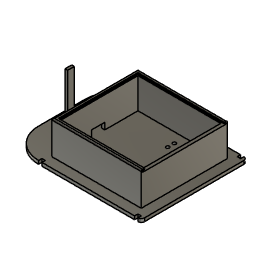
Robot_body (Autodesk Fusion 360 design; units mm, degrees)
Autodesk Fusion 360 part; units mm, degrees
sketch "Szkic1" plane through (0, 0, 0) normal (0, 0, 1) x (1, 0, 0)
  line L0 (100, -80) -> (-100, -80)
  line L1 (-100, -80) -> (-100, 80)
  line L2 (-100, 80) -> (100, 80)
  line L3 (100, 80) -> (100, -80)
  line L4 (100, -80) -> (-100, 80) construction
  line L5 (-100, -80) -> (100, 80) construction
  dimension "d1" = 200
  dimension "d2" = 160
  constraint horizontal L0
  constraint perpendicular L0 L1
  constraint parallel L0 L2
  constraint parallel L1 L3
  constraint coincident L4 origin
  constraint coincident L5 origin
  measures "d1" distance of L1.end L2.end
  measures "d2" distance of L0.end L1.end
extrude "Wyciągnięcie proste1" add sketch "Szkic1" along normal blind 5
sketch "Szkic2" plane through (0, 0, 5) normal (0, 0, 1) x (-1, 0, 0)
  line L0 (-100, -80) -> (100, -80)
  line L1 (100, -80) -> (100, 80)
  line L2 (100, 80) -> (-100, 80)
  line L3 (-100, 80) -> (-100, -80)
  line L4 (-90, 80) -> (-95, 80)
  line L5 (-95, 80) -> (-95, 75)
  line L6 (-95, 75) -> (-90, 75)
  line L7 (-90, 75) -> (-90, 80)
  dimension "d5" = 5
  dimension "d6" = 5
  constraint horizontal L4
  constraint vertical L5
  constraint horizontal L6
  constraint vertical L7
  constraint coincident L2 L4.start
  measures "d5" distance of L4.start L4.end
  measures "d6" distance of L4.start L6.end
extrude "Wyciągnięcie proste2" cut sketch "Szkic2" against normal blind 5 contours L2 L4 L5 L6 L7
sketch "Szkic3" plane through (0, 0, 5) normal (0, 0, 1) x (-1, 0, 0)
  line L0 (-95, 75) -> (-95, 80)
  line L1 (-95, 80) -> (-100, 80)
  line L2 (-100, 80) -> (-100, -80)
  line L3 (-100, -80) -> (100, -80)
  line L4 (100, -80) -> (100, 80)
  line L5 (100, 80) -> (-90, 80)
  line L6 (-90, 80) -> (-90, 75)
  line L7 (-90, 75) -> (-95, 75)
  line L8 (-90, -80) -> (-95, -80)
  line L9 (-95, -80) -> (-95, -75)
  line L10 (-95, -75) -> (-90, -75)
  line L11 (-90, -75) -> (-90, -80)
  dimension "d9" = 5
  dimension "d10" = 5
  constraint horizontal L8
  constraint vertical L9
  constraint horizontal L10
  constraint vertical L11
  constraint coincident L3 L8.start
  measures "d9" distance of L8.start L8.end
  measures "d10" distance of L8.start L10.end
extrude "Wyciągnięcie proste3" cut sketch "Szkic3" against normal blind 5 contours L3 L8 L9 L10 L11
sketch "Szkic4" plane through (0, 0, 5) normal (0, 0, 1) x (-1, 0, 0)
  line L0 (-90, -75) -> (-90, -80)
  line L1 (-90, -80) -> (100, -80)
  line L2 (100, -80) -> (100, 80)
  line L3 (100, 80) -> (-90, 80)
  line L4 (-90, 80) -> (-90, 75)
  line L5 (-90, 75) -> (-95, 75)
  line L6 (-95, 75) -> (-95, 80)
  line L7 (-95, 80) -> (-100, 80)
  line L8 (-100, 80) -> (-100, -80)
  line L9 (-100, -80) -> (-95, -80)
  line L10 (-95, -80) -> (-95, -75)
  line L11 (-95, -75) -> (-90, -75)
  line L12 (50, -80) -> (55, -80)
  line L13 (55, -80) -> (55, -75)
  line L14 (55, -75) -> (50, -75)
  line L15 (50, -75) -> (50, -80)
  dimension "d13" = 5
  dimension "d14" = 5
  constraint horizontal L12
  constraint vertical L13
  constraint horizontal L14
  constraint vertical L15
  constraint coincident L1 L12.start
  measures "d13" distance of L12.start L12.end
  measures "d14" distance of L12.start L14.end
extrude "Wyciągnięcie proste4" cut sketch "Szkic4" against normal blind 5 contours L1 L12 L13 L14 L15
sketch "Szkic5" plane through (0, 0, 5) normal (0, 0, 1) x (-1, 0, 0)
  line L0 (50, -80) -> (50, -75)
  line L1 (50, -75) -> (55, -75)
  line L2 (55, -75) -> (55, -80)
  line L3 (55, -80) -> (100, -80)
  line L4 (100, -80) -> (100, 80)
  line L5 (100, 80) -> (-90, 80)
  line L6 (-90, 80) -> (-90, 75)
  line L7 (-90, 75) -> (-95, 75)
  line L8 (-95, 75) -> (-95, 80)
  line L9 (-95, 80) -> (-100, 80)
  line L10 (-100, 80) -> (-100, -80)
  line L11 (-100, -80) -> (-95, -80)
  line L12 (-95, -80) -> (-95, -75)
  line L13 (-95, -75) -> (-90, -75)
  line L14 (-90, -75) -> (-90, -80)
  line L15 (-90, -80) -> (50, -80)
  line L16 (50, 80) -> (55, 80)
  line L17 (55, 80) -> (55, 75)
  line L18 (55, 75) -> (50, 75)
  line L19 (50, 75) -> (50, 80)
  dimension "d17" = 5
  dimension "d18" = 5
  constraint horizontal L16
  constraint vertical L17
  constraint horizontal L18
  constraint vertical L19
  constraint coincident L5 L16.start
  measures "d17" distance of L16.start L16.end
  measures "d18" distance of L16.start L18.end
extrude "Wyciągnięcie proste5" cut sketch "Szkic5" against normal blind 5 contours L5 L16 L17 L18 L19
sketch "Szkic6" plane through (0, 0, 5) normal (0, 0, 1) x (-1, 0, 0)
  line L0 (50, 75) -> (50, 80)
  line L1 (50, 80) -> (-90, 80)
  line L2 (-90, 80) -> (-90, 75)
  line L3 (-90, 75) -> (-95, 75)
  line L4 (-95, 75) -> (-95, 80)
  line L5 (-95, 80) -> (-100, 80)
  line L6 (-100, 80) -> (-100, -80)
  line L7 (-100, -80) -> (-95, -80)
  line L8 (-95, -80) -> (-95, -75)
  line L9 (-95, -75) -> (-90, -75)
  line L10 (-90, -75) -> (-90, -80)
  line L11 (-90, -80) -> (50, -80)
  line L12 (50, -80) -> (50, -75)
  line L13 (50, -75) -> (55, -75)
  line L14 (55, -75) -> (55, -80)
  line L15 (55, -80) -> (100, -80)
  line L16 (100, -80) -> (100, 80)
  line L17 (100, 80) -> (55, 80)
  line L18 (55, 80) -> (55, 75)
  line L19 (55, 75) -> (50, 75)
  line L20 (50, -65) -> (45, -65)
  line L21 (45, -65) -> (45, 65)
  line L22 (45, 65) -> (50, 65)
  line L23 (50, 65) -> (50, -65)
  constraint horizontal L20
  constraint vertical L21
  constraint horizontal L22
  constraint vertical L23
extrude "Wyciągnięcie proste6" add sketch "Szkic6" along normal blind 50 contours L20 L21 L22 L23
sketch "Szkic7" plane through (-45, 0, 0) normal (1, 0, 0) x (0, 1, 0)
  line L0 (-65, 5) -> (65, 5)
  line L1 (65, 5) -> (65, 55)
  line L2 (65, 55) -> (-65, 55)
  line L3 (-65, 55) -> (-65, 5)
  line L4 (-63, 53) -> (63, 53)
  line L5 (63, 53) -> (63, 51)
  line L6 (63, 51) -> (-63, 51)
  line L7 (-63, 51) -> (-63, 53)
  constraint horizontal L4
  constraint vertical L5
  constraint horizontal L6
  constraint vertical L7
extrude "Wyciągnięcie proste7" cut sketch "Szkic7" against normal blind 2 contours L4 L5 L6 L7
sketch "Szkic8" plane through (0, 0, 5) normal (0, 0, 1) x (-1, 0, 0)
  line L0 (50, 65) -> (50, -65)
  line L1 (50, -65) -> (45, -65)
  line L2 (45, -65) -> (45, 65)
  line L3 (45, 65) -> (50, 65)
  line L4 (50, 75) -> (50, 80)
  line L5 (50, 80) -> (-90, 80)
  line L6 (-90, 80) -> (-90, 75)
  line L7 (-90, 75) -> (-95, 75)
  line L8 (-95, 75) -> (-95, 80)
  line L9 (-95, 80) -> (-100, 80)
  line L10 (-100, 80) -> (-100, -80)
  line L11 (-100, -80) -> (-95, -80)
  line L12 (-95, -80) -> (-95, -75)
  line L13 (-95, -75) -> (-90, -75)
  line L14 (-90, -75) -> (-90, -80)
  line L15 (-90, -80) -> (50, -80)
  line L16 (50, -80) -> (50, -75)
  line L17 (50, -75) -> (55, -75)
  line L18 (55, -75) -> (55, -80)
  line L19 (55, -80) -> (100, -80)
  line L20 (100, -80) -> (100, 80)
  line L21 (100, 80) -> (55, 80)
  line L22 (55, 80) -> (55, 75)
  line L23 (55, 75) -> (50, 75)
  line L24 (45, 65) -> (-85, 65)
  line L25 (-85, 65) -> (-85, 60)
  line L26 (-85, 60) -> (45, 60)
  line L27 (45, 60) -> (45, 65)
  dimension "d25" = 130
  constraint horizontal L24
  constraint vertical L25
  constraint horizontal L26
  constraint vertical L27
  constraint coincident L2.end L3.start
  measures "d25" distance of L2.end L24.end
extrude "Wyciągnięcie proste8" add sketch "Szkic8" along normal blind 50 contours L2 L24 L25 L26 L27
sketch "Szkic9" plane through (0, -60, 0) normal (0, 1, 0) x (-1, 0, 0)
  line L0 (-85, 5) -> (45, 5)
  line L1 (45, 5) -> (45, 51)
  line L2 (45, 51) -> (45, 53)
  line L3 (45, 53) -> (45, 55)
  line L4 (45, 55) -> (-85, 55)
  line L5 (-85, 55) -> (-85, 5)
  line L6 (-85, 53) -> (45, 53)
  line L7 (45, 53) -> (45, 51)
  line L8 (45, 51) -> (-85, 51)
  line L9 (-85, 51) -> (-85, 53)
  constraint horizontal L6
  constraint vertical L7
  constraint horizontal L8
  constraint vertical L9
  constraint coincident L1.end L2.start
  constraint coincident L5 L6.start
extrude "Wyciągnięcie proste9" cut sketch "Szkic9" against normal blind 3 contours L2 L5 L6 L7 L8 L9
sketch "Szkic10" plane through (0, 0, 5) normal (0, 0, 1) x (-1, 0, 0)
  line L0 (50, 75) -> (50, 80)
  line L1 (50, 80) -> (-90, 80)
  line L2 (-90, 80) -> (-90, 75)
  line L3 (-90, 75) -> (-95, 75)
  line L4 (-95, 75) -> (-95, 80)
  line L5 (-95, 80) -> (-100, 80)
  line L6 (-100, 80) -> (-100, -80)
  line L7 (-100, -80) -> (-95, -80)
  line L8 (-95, -80) -> (-95, -75)
  line L9 (-95, -75) -> (-90, -75)
  line L10 (-90, -75) -> (-90, -80)
  line L11 (-90, -80) -> (50, -80)
  line L12 (50, -80) -> (50, -75)
  line L13 (50, -75) -> (55, -75)
  line L14 (55, -75) -> (55, -80)
  line L15 (55, -80) -> (100, -80)
  line L16 (100, -80) -> (100, 80)
  line L17 (100, 80) -> (55, 80)
  line L18 (55, 80) -> (55, 75)
  line L19 (55, 75) -> (50, 75)
  line L20 (45, 60) -> (-85, 60)
  line L21 (-85, 60) -> (-85, 65)
  line L22 (-85, 65) -> (50, 65)
  line L23 (50, 65) -> (50, -65)
  line L24 (50, -65) -> (45, -65)
  line L25 (45, -65) -> (45, 60)
  line L26 (45, -65) -> (-85, -65)
  line L27 (-85, -65) -> (-85, -60)
  line L28 (-85, -60) -> (45, -60)
  line L29 (45, -60) -> (45, -65)
  constraint horizontal L26
  constraint vertical L27
  constraint horizontal L28
  constraint vertical L29
  constraint coincident L24.end L25.start
extrude "Wyciągnięcie proste10" add sketch "Szkic10" along normal blind 50 contours L25 L26 L27 L28 L29
sketch "Szkic11" plane through (85, 0, 0) normal (1, 0, 0) x (0, 1, 0)
  line L0 (60, 5) -> (65, 5)
  line L1 (65, 5) -> (65, 55)
  line L2 (65, 55) -> (60, 55)
  line L3 (60, 55) -> (60, 5)
  line L4 (60, 53) -> (63, 53)
  line L5 (63, 53) -> (63, 51)
  line L6 (63, 51) -> (60, 51)
  line L7 (60, 51) -> (60, 53)
  constraint horizontal L4
  constraint vertical L5
  constraint horizontal L6
  constraint vertical L7
  constraint coincident L3 L4.start
extrude "Wyciągnięcie proste11" cut sketch "Szkic11" against normal blind 130 contours L3 L4 L5 L6 L7
sketch "Szkic12" plane through (0, 0, 5) normal (0, 0, 1) x (-1, 0, 0)
  line L0 (50, -65) -> (-85, -65)
  line L1 (-85, -65) -> (-85, -60)
  line L2 (-85, -60) -> (45, -60)
  line L3 (45, -60) -> (45, 60)
  line L4 (45, 60) -> (-85, 60)
  line L5 (-85, 60) -> (-85, 65)
  line L6 (-85, 65) -> (50, 65)
  line L7 (50, 65) -> (50, -65)
  line L8 (50, 75) -> (50, 80)
  line L9 (50, 80) -> (-90, 80)
  line L10 (-90, 80) -> (-90, 75)
  line L11 (-90, 75) -> (-95, 75)
  line L12 (-95, 75) -> (-95, 80)
  line L13 (-95, 80) -> (-100, 80)
  line L14 (-100, 80) -> (-100, -80)
  line L15 (-100, -80) -> (-95, -80)
  line L16 (-95, -80) -> (-95, -75)
  line L17 (-95, -75) -> (-90, -75)
  line L18 (-90, -75) -> (-90, -80)
  line L19 (-90, -80) -> (50, -80)
  line L20 (50, -80) -> (50, -75)
  line L21 (50, -75) -> (55, -75)
  line L22 (55, -75) -> (55, -80)
  line L23 (55, -80) -> (100, -80)
  line L24 (100, -80) -> (100, 80)
  line L25 (100, 80) -> (55, 80)
  line L26 (55, 80) -> (55, 75)
  line L27 (55, 75) -> (50, 75)
  line L28 (-85, 60) -> (-80, 60)
  line L29 (-80, 60) -> (-80, -60)
  line L30 (-80, -60) -> (-85, -60)
  line L31 (-85, -60) -> (-85, 60)
  constraint horizontal L28
  constraint vertical L29
  constraint horizontal L30
  constraint vertical L31
  constraint coincident L2 L29.end
  constraint coincident L4.end L5.start
extrude "Wyciągnięcie proste12" add sketch "Szkic12" along normal blind 46 contours L2 L4 L28 L29 L30 L31
sketch "Szkic13" plane through (0, 0, 5) normal (0, 0, 1) x (-1, 0, 0)
  line L0 (-80, 60) -> (-80, -60)
  line L1 (-80, -60) -> (45, -60)
  line L2 (45, -60) -> (45, 60)
  line L3 (45, 60) -> (-80, 60)
  circle A0 centre (-25, -45) radius 2.5
  dimension "d36" = 5
  measures "d36" diameter of A0
extrude "Wyciągnięcie proste13" cut sketch "Szkic13" against normal blind 5 contours A0
sketch "Szkic14" plane through (0, 0, 5) normal (0, 0, 1) x (-1, 0, 0)
  circle A0 centre (-25, -45) radius 2.5
  line L0 (-80, 60) -> (-80, -60)
  line L1 (-80, -60) -> (45, -60)
  line L2 (45, -60) -> (45, 60)
  line L3 (45, 60) -> (-80, 60)
  circle A1 centre (-25, -35) radius 2.5
  dimension "d39" = 5
  measures "d39" diameter of A1
extrude "Wyciągnięcie proste14" cut sketch "Szkic14" against normal blind 5 contours A1
sketch "Szkic15" plane through (0, 0, 5) normal (0, 0, 1) x (-1, 0, 0)
  circle A0 centre (-25, -35) radius 2.5
  circle A1 centre (-25, -45) radius 2.5
  line L0 (-80, 60) -> (-80, -60)
  line L1 (-80, -60) -> (45, -60)
  line L2 (45, -60) -> (45, 60)
  line L3 (45, 60) -> (-80, 60)
  circle A2 centre (-25, 35) radius 2.5
  dimension "d42" = 5
  measures "d42" diameter of A2
extrude "Wyciągnięcie proste15" cut sketch "Szkic15" against normal blind 5 contours A2
sketch "Szkic16" plane through (0, 0, 5) normal (0, 0, 1) x (-1, 0, 0)
  circle A0 centre (-25, 35) radius 2.5
  circle A1 centre (-25, -35) radius 2.5
  circle A2 centre (-25, -45) radius 2.5
  line L0 (-80, 60) -> (-80, -60)
  line L1 (-80, -60) -> (45, -60)
  line L2 (45, -60) -> (45, 60)
  line L3 (45, 60) -> (-80, 60)
  circle A3 centre (-25, 45) radius 2.5
  dimension "d45" = 5
  measures "d45" diameter of A3
extrude "Wyciągnięcie proste16" cut sketch "Szkic16" against normal blind 5 contours A3
sketch "Szkic17" plane through (0, 0, 5) normal (0, 0, 1) x (-1, 0, 0)
  line L0 (-85, -65) -> (-85, 65)
  line L1 (-85, 65) -> (50, 65)
  line L2 (50, 65) -> (50, -65)
  line L3 (50, -65) -> (-85, -65)
  line L4 (50, 75) -> (50, 80)
  line L5 (50, 80) -> (-90, 80)
  line L6 (-90, 80) -> (-90, 75)
  line L7 (-90, 75) -> (-95, 75)
  line L8 (-95, 75) -> (-95, 80)
  line L9 (-95, 80) -> (-100, 80)
  line L10 (-100, 80) -> (-100, -80)
  line L11 (-100, -80) -> (-95, -80)
  line L12 (-95, -80) -> (-95, -75)
  line L13 (-95, -75) -> (-90, -75)
  line L14 (-90, -75) -> (-90, -80)
  line L15 (-90, -80) -> (50, -80)
  line L16 (50, -80) -> (50, -75)
  line L17 (50, -75) -> (55, -75)
  line L18 (55, -75) -> (55, -80)
  line L19 (55, -80) -> (100, -80)
  line L20 (100, -80) -> (100, 80)
  line L21 (100, 80) -> (55, 80)
  line L22 (55, 80) -> (55, 75)
  line L23 (55, 75) -> (50, 75)
  line L24 (55, -80) -> (55, -35)
  line L25 (55, -35) -> (100, -35)
  arc A0 (55, -80) -> (100, -35) centre (55, -35) ccw
  point P0 (100, -80)
  dimension "d48" = 45
  dimension "d49" = 45
  dimension "d50" = 45
  constraint vertical L24
  constraint horizontal L25
  constraint coincident P0 L19.end
  constraint coincident L18.end L19.start
  constraint coincident L25.end A0.end
  measures "d48" distance of P0 L18.end
  measures "d49" distance of P0 L25.end
  measures "d50" radius of A0
extrude "Wyciągnięcie proste17" cut sketch "Szkic17" against normal blind 5 contours L19 L20 A0
sketch "Szkic18" plane through (0, 0, 5) normal (0, 0, 1) x (-1, 0, 0)
  arc A0 (55, -80) -> (100, -35) centre (55, -35) ccw
  line L0 (100, -35) -> (100, 80)
  line L1 (100, 80) -> (55, 80)
  line L2 (55, 80) -> (55, 75)
  line L3 (55, 75) -> (50, 75)
  line L4 (50, 75) -> (50, 80)
  line L5 (50, 80) -> (-90, 80)
  line L6 (-90, 80) -> (-90, 75)
  line L7 (-90, 75) -> (-95, 75)
  line L8 (-95, 75) -> (-95, 80)
  line L9 (-95, 80) -> (-100, 80)
  line L10 (-100, 80) -> (-100, -80)
  line L11 (-100, -80) -> (-95, -80)
  line L12 (-95, -80) -> (-95, -75)
  line L13 (-95, -75) -> (-90, -75)
  line L14 (-90, -75) -> (-90, -80)
  line L15 (-90, -80) -> (50, -80)
  line L16 (50, -80) -> (50, -75)
  line L17 (50, -75) -> (55, -75)
  line L18 (55, -75) -> (55, -80)
  line L19 (-85, -65) -> (-85, 65)
  line L20 (-85, 65) -> (50, 65)
  line L21 (50, 65) -> (50, -65)
  line L22 (50, -65) -> (-85, -65)
  line L23 (55, 80) -> (55, 35)
  line L24 (55, 35) -> (100, 35)
  arc A1 (100, 35) -> (55, 80) centre (55, 35) ccw
  point P0 (100, 80)
  dimension "d53" = 45
  dimension "d54" = 45
  dimension "d55" = 45
  constraint vertical L23
  constraint horizontal L24
  constraint coincident P0 L0.end
  constraint coincident L1.end L2.start
  constraint coincident L24.end A1.start
  measures "d53" distance of P0 L1.end
  measures "d54" distance of P0 L24.end
  measures "d55" radius of A1
extrude "Wyciągnięcie proste18" cut sketch "Szkic18" against normal blind 5 contours L0 L1 A1
sketch "Szkic19" plane through (0, 0, 5) normal (0, 0, 1) x (-1, 0, 0)
  arc A0 (100, 35) -> (55, 80) centre (55, 35) ccw
  line L0 (55, 80) -> (55, 75)
  line L1 (55, 75) -> (50, 75)
  line L2 (50, 75) -> (50, 80)
  line L3 (50, 80) -> (-90, 80)
  line L4 (-90, 80) -> (-90, 75)
  line L5 (-90, 75) -> (-95, 75)
  line L6 (-95, 75) -> (-95, 80)
  line L7 (-95, 80) -> (-100, 80)
  line L8 (-100, 80) -> (-100, -80)
  line L9 (-100, -80) -> (-95, -80)
  line L10 (-95, -80) -> (-95, -75)
  line L11 (-95, -75) -> (-90, -75)
  line L12 (-90, -75) -> (-90, -80)
  line L13 (-90, -80) -> (50, -80)
  line L14 (50, -80) -> (50, -75)
  line L15 (50, -75) -> (55, -75)
  line L16 (55, -75) -> (55, -80)
  arc A1 (55, -80) -> (100, -35) centre (55, -35) ccw
  line L17 (100, -35) -> (100, 35)
  line L18 (-85, -65) -> (-85, 65)
  line L19 (-85, 65) -> (50, 65)
  line L20 (50, 65) -> (50, -65)
  line L21 (50, -65) -> (-85, -65)
  line L22 (-100, -75) -> (-95, -75)
  line L23 (-95, -75) -> (-95, -80)
  arc A2 (-100, -75) -> (-95, -80) centre (-95, -75) ccw
  dimension "d58" = 5
  constraint horizontal L22
  constraint vertical L23
  constraint coincident L8 L22.start
  constraint coincident L9.end L10.start
  constraint coincident L22.start A2.start
  measures "d58" radius of A2
extrude "Wyciągnięcie proste19" cut sketch "Szkic19" against normal blind 5 contours L8 L9 A2
sketch "Szkic20" plane through (0, 0, 5) normal (0, 0, 1) x (-1, 0, 0)
  arc A0 (-100, -75) -> (-95, -80) centre (-95, -75) ccw
  line L0 (-95, -80) -> (-95, -75)
  line L1 (-95, -75) -> (-90, -75)
  line L2 (-90, -75) -> (-90, -80)
  line L3 (-90, -80) -> (50, -80)
  line L4 (50, -80) -> (50, -75)
  line L5 (50, -75) -> (55, -75)
  line L6 (55, -75) -> (55, -80)
  arc A1 (55, -80) -> (100, -35) centre (55, -35) ccw
  line L7 (100, -35) -> (100, 35)
  arc A2 (100, 35) -> (55, 80) centre (55, 35) ccw
  line L8 (55, 80) -> (55, 75)
  line L9 (55, 75) -> (50, 75)
  line L10 (50, 75) -> (50, 80)
  line L11 (50, 80) -> (-90, 80)
  line L12 (-90, 80) -> (-90, 75)
  line L13 (-90, 75) -> (-95, 75)
  line L14 (-95, 75) -> (-95, 80)
  line L15 (-95, 80) -> (-100, 80)
  line L16 (-100, 80) -> (-100, -75)
  line L17 (-85, -65) -> (-85, 65)
  line L18 (-85, 65) -> (50, 65)
  line L19 (50, 65) -> (50, -65)
  line L20 (50, -65) -> (-85, -65)
  line L21 (-100, 75) -> (-95, 75)
  line L22 (-95, 75) -> (-95, 80)
  arc A3 (-95, 80) -> (-100, 75) centre (-95, 75) ccw
  dimension "d61" = 5
  constraint horizontal L21
  constraint vertical L22
  constraint coincident L16 L21.start
  constraint coincident L14.end L15.start
  constraint coincident L21.start A3.end
  measures "d61" radius of A3
extrude "Wyciągnięcie proste20" cut sketch "Szkic20" against normal blind 5 contours L15 L16 A3
sketch "Szkic21" plane through (-50, 0, 0) normal (-1, 0, 0) x (0, -1, 0)
  line L0 (-65, 5) -> (65, 5)
  line L1 (65, 5) -> (65, 55)
  line L2 (65, 55) -> (-65, 55)
  line L3 (-65, 55) -> (-65, 5)
  line L4 (0, 5) -> (10, 5)
  line L5 (10, 5) -> (10, 15)
  line L6 (10, 15) -> (0, 15)
  line L7 (0, 15) -> (0, 5)
  dimension "d64" = 10
  dimension "d65" = 10
  constraint horizontal L4
  constraint vertical L5
  constraint horizontal L6
  constraint vertical L7
  constraint midpoint L0 L4.start
  measures "d64" distance of L4.start L4.end
  measures "d65" distance of L4.start L6.end
extrude "Wyciągnięcie proste21" cut sketch "Szkic21" against normal blind 5 contours L0 L4 L5 L6 L7
sketch "Szkic22" plane through (-50, 0, 0) normal (-1, 0, 0) x (0, -1, 0)
  line L0 (0, 5) -> (0, 15)
  line L1 (0, 15) -> (10, 15)
  line L2 (10, 15) -> (10, 5)
  line L3 (10, 5) -> (65, 5)
  line L4 (65, 5) -> (65, 55)
  line L5 (65, 55) -> (-65, 55)
  line L6 (-65, 55) -> (-65, 5)
  line L7 (-65, 5) -> (0, 5)
  line L8 (0, 5) -> (-10, 5)
  line L9 (-10, 5) -> (-10, 15)
  line L10 (-10, 15) -> (0, 15)
  line L11 (0, 15) -> (0, 5)
  dimension "d68" = 10
  dimension "d69" = 10
  constraint horizontal L8
  constraint vertical L9
  constraint horizontal L10
  constraint vertical L11
  constraint coincident L0.start L7.end
  measures "d68" distance of L0.start L8.end
  measures "d69" distance of L0.start L0.end
extrude "Wyciągnięcie proste22" cut sketch "Szkic22" against normal blind 5 contours L0 L7 L8 L9 L10 L11
sketch "Szkic23" plane through (0, 0, 5) normal (0, 0, 1) x (-1, 0, 0)
  arc A0 (-95, 80) -> (-100, 75) centre (-95, 75) ccw
  line L0 (-100, 75) -> (-100, -75)
  arc A1 (-100, -75) -> (-95, -80) centre (-95, -75) ccw
  line L1 (-95, -80) -> (-95, -75)
  line L2 (-95, -75) -> (-90, -75)
  line L3 (-90, -75) -> (-90, -80)
  line L4 (-90, -80) -> (50, -80)
  line L5 (50, -80) -> (50, -75)
  line L6 (50, -75) -> (55, -75)
  line L7 (55, -75) -> (55, -80)
  arc A2 (55, -80) -> (100, -35) centre (55, -35) ccw
  line L8 (100, -35) -> (100, 35)
  arc A3 (100, 35) -> (55, 80) centre (55, 35) ccw
  line L9 (55, 80) -> (55, 75)
  line L10 (55, 75) -> (50, 75)
  line L11 (50, 75) -> (50, 80)
  line L12 (50, 80) -> (-90, 80)
  line L13 (-90, 80) -> (-90, 75)
  line L14 (-90, 75) -> (-95, 75)
  line L15 (-95, 75) -> (-95, 80)
  circle A4 centre (-25, 45) radius 2.5
  circle A5 centre (-25, 35) radius 2.5
  circle A6 centre (-25, -35) radius 2.5
  circle A7 centre (-25, -45) radius 2.5
  line L16 (-80, 60) -> (-80, -60)
  line L17 (-80, -60) -> (45, -60)
  line L18 (45, -60) -> (45, -10)
  line L19 (45, -10) -> (50, -10)
  line L20 (50, -10) -> (50, -65)
  line L21 (50, -65) -> (-85, -65)
  line L22 (-85, -65) -> (-85, 65)
  line L23 (-85, 65) -> (50, 65)
  line L24 (50, 65) -> (50, 10)
  line L25 (50, 10) -> (45, 10)
  line L26 (45, 10) -> (45, 60)
  line L27 (45, 60) -> (-80, 60)
  line L28 (75.3615, 5.2617) -> (80.3615, 5.2617)
  line L29 (80.3615, 5.2617) -> (80.3615, -4.7383)
  line L30 (80.3615, -4.7383) -> (75.3615, -4.7383)
  line L31 (75.3615, -4.7383) -> (75.3615, 5.2617)
  dimension "d72" = 5
  dimension "d73" = 10
  constraint horizontal L28
  constraint vertical L29
  constraint horizontal L30
  constraint vertical L31
  measures "d72" distance of L28.start L28.end
  measures "d73" distance of L28.start L30.end
extrude "Wyciągnięcie proste23" add sketch "Szkic23" along normal blind 50 contours L28 L29 L30 L31
sketch "Szkic24" plane through (-80.3615, 0, 0) normal (-1, 0, 0) x (0, -1, 0)
  line L0 (-4.7383, 5) -> (5.2617, 5)
  line L1 (5.2617, 5) -> (5.2617, 55)
  line L2 (5.2617, 55) -> (-4.7383, 55)
  line L3 (-4.7383, 55) -> (-4.7383, 5)
  line L4 (-4.7383, 55) -> (5.2617, 55)
  line L5 (5.2617, 55) -> (5.2617, 45)
  line L6 (5.2617, 45) -> (-4.7383, 45)
  line L7 (-4.7383, 45) -> (-4.7383, 55)
  dimension "d76" = 10
  dimension "d77" = 10
  constraint horizontal L4
  constraint vertical L5
  constraint horizontal L6
  constraint vertical L7
  constraint coincident L2.end L3.start
  measures "d76" distance of L2.end L1.end
  measures "d77" distance of L2.end L6.end
extrude "Wyciągnięcie proste24" add sketch "Szkic24" along normal blind 10 contours L1 L2 L3 L4 L5 L6 L7
sketch "Szkic25" plane through (0, -5.2617, 0) normal (0, -1, 0) x (1, 0, 0)
  line L0 (-80.3615, 5) -> (-75.3615, 5)
  line L1 (-75.3615, 5) -> (-75.3615, 55)
  line L2 (-75.3615, 55) -> (-90.3615, 55)
  line L3 (-90.3615, 55) -> (-90.3615, 45)
  line L4 (-90.3615, 45) -> (-80.3615, 45)
  line L5 (-80.3615, 45) -> (-80.3615, 5)
  line L6 (-90.3615, 45) -> (-80, 55)
  constraint coincident L3.end L4.start
  constraint coincident L2 L6.end
extrude "Wyciągnięcie proste25" cut sketch "Szkic25" against normal blind 10 contours L2 L3 L6
sketch "Szkic26" plane through (0, -5.2617, 0) normal (0, -1, 0) x (1, 0, 0)
  line L0 (-80, 55) -> (-90.3615, 45)
  line L1 (-90.3615, 45) -> (-80.3615, 45)
  line L2 (-80.3615, 45) -> (-80.3615, 5)
  line L3 (-80.3615, 5) -> (-75.3615, 5)
  line L4 (-75.3615, 5) -> (-75.3615, 55)
  line L5 (-75.3615, 55) -> (-80, 55)
  line L6 (-80, 55) -> (-85.3615, 45)
  constraint coincident L0.start L5.end
  constraint midpoint L1 L6.end
extrude "Wyciągnięcie proste26" cut sketch "Szkic26" against normal blind 10 contours L0 L1 L6
sketch "Szkic27" plane through (85, 0, 0) normal (1, 0, 0) x (0, 1, 0)
  line L0 (-63, 53) -> (-60, 53)
  line L1 (-60, 53) -> (-60, 55)
  line L2 (-60, 55) -> (-65, 55)
  line L3 (-65, 55) -> (-65, 5)
  line L4 (-65, 5) -> (65, 5)
  line L5 (65, 5) -> (65, 55)
  line L6 (65, 55) -> (60, 55)
  line L7 (60, 55) -> (60, 53)
  line L8 (60, 53) -> (63, 53)
  line L9 (63, 53) -> (63, 51)
  line L10 (63, 51) -> (-63, 51)
  line L11 (-63, 51) -> (-63, 53)
  line L12 (63, 53) -> (65, 53)
  line L13 (63, 55) -> (63, 53)
  arc A0 (65, 53) -> (63, 55) centre (63, 53) ccw
  dimension "d84" = 2
  constraint horizontal L12
  constraint vertical L13
  constraint coincident L8.end L9.start
  constraint coincident L12.end A0.start
  constraint coincident L13.start A0.end
  measures "d84" radius of A0
extrude "Wyciągnięcie proste27" cut sketch "Szkic27" against normal blind 140 contours L5 L6 A0
sketch "Szkic28" plane through (0, -65, 0) normal (0, -1, 0) x (1, 0, 0)
  line L0 (-50, 5) -> (85, 5)
  line L1 (85, 5) -> (85, 55)
  line L2 (85, 55) -> (-50, 55)
  line L3 (-50, 55) -> (-50, 5)
  line L4 (-50, 53) -> (-48, 53)
  line L5 (-48, 53) -> (-48, 55)
  arc A0 (-48, 55) -> (-50, 53) centre (-48, 53) ccw
  dimension "d87" = 2
  constraint horizontal L4
  constraint vertical L5
  constraint coincident L2 L5.end
  constraint coincident L3 L4.start
  constraint coincident L5.end A0.start
  constraint coincident L4.start A0.end
  measures "d87" radius of A0
extrude "Wyciągnięcie proste28" cut sketch "Szkic28" against normal blind 140 contours L2 L3 A0
sketch "Szkic29" plane through (85, 0, 0) normal (1, 0, 0) x (0, 1, 0)
  arc A0 (65, 53) -> (63, 55) centre (63, 53) ccw
  line L0 (63, 55) -> (60, 55)
  line L1 (60, 55) -> (60, 53)
  line L2 (60, 53) -> (63, 53)
  line L3 (63, 53) -> (63, 51)
  line L4 (63, 51) -> (-63, 51)
  line L5 (-63, 51) -> (-63, 53)
  line L6 (-63, 53) -> (-60, 53)
  line L7 (-60, 53) -> (-60, 55)
  line L8 (-60, 55) -> (-65, 55)
  line L9 (-65, 55) -> (-65, 5)
  line L10 (-65, 5) -> (65, 5)
  line L11 (65, 5) -> (65, 53)
  line L12 (-63, 55) -> (-63, 53)
  line L13 (-63, 53) -> (-65, 53)
  arc A1 (-63, 55) -> (-65, 53) centre (-63, 53) ccw
  dimension "d90" = 2
  constraint vertical L12
  constraint horizontal L13
  constraint coincident L5.end L6.start
  constraint coincident L12.start A1.start
  constraint coincident L13.end A1.end
  measures "d90" radius of A1
extrude "Wyciągnięcie proste29" cut sketch "Szkic29" against normal blind 140 contours L8 L9 A1
sketch "Sketch30" plane through (0, 0, 5) normal (0, 0, 1) x (-1, 0, 0)
  line L0 (75.3615, -4.7383) -> (75.3615, 5.2617)
  line L1 (75.3615, 5.2617) -> (80.3615, 5.2617)
  line L2 (80.3615, 5.2617) -> (80.3615, -4.7383)
  line L3 (80.3615, -4.7383) -> (75.3615, -4.7383)
  arc A0 (-95, 80) -> (-100, 75) centre (-95, 75) ccw
  line L4 (-100, 75) -> (-100, -75)
  arc A1 (-100, -75) -> (-95, -80) centre (-95, -75) ccw
  line L5 (-95, -80) -> (-95, -75)
  line L6 (-95, -75) -> (-90, -75)
  line L7 (-90, -75) -> (-90, -80)
  line L8 (-90, -80) -> (50, -80)
  line L9 (50, -80) -> (50, -75)
  line L10 (50, -75) -> (55, -75)
  line L11 (55, -75) -> (55, -80)
  arc A2 (55, -80) -> (100, -35) centre (55, -35) ccw
  line L12 (100, -35) -> (100, 35)
  arc A3 (100, 35) -> (55, 80) centre (55, 35) ccw
  line L13 (55, 80) -> (55, 75)
  line L14 (55, 75) -> (50, 75)
  line L15 (50, 75) -> (50, 80)
  line L16 (50, 80) -> (-90, 80)
  line L17 (-90, 80) -> (-90, 75)
  line L18 (-90, 75) -> (-95, 75)
  line L19 (-95, 75) -> (-95, 80)
  circle A4 centre (-25, 45) radius 2.5
  circle A5 centre (-25, 35) radius 2.5
  circle A6 centre (-25, -35) radius 2.5
  circle A7 centre (-25, -45) radius 2.5
  line L20 (-80, 60) -> (-80, -60)
  line L21 (-80, -60) -> (45, -60)
  line L22 (45, -60) -> (45, -10)
  line L23 (45, -10) -> (50, -10)
  line L24 (50, -10) -> (50, -65)
  line L25 (50, -65) -> (-85, -65)
  line L26 (-85, -65) -> (-85, 65)
  line L27 (-85, 65) -> (50, 65)
  line L28 (50, 65) -> (50, 10)
  line L29 (50, 10) -> (45, 10)
  line L30 (45, 10) -> (45, 60)
  line L31 (45, 60) -> (-80, 60)
  line L32 (90, -30) -> (80, -30)
  line L33 (80, -30) -> (80, -20)
  line L34 (80, -20) -> (90, -20)
  line L35 (90, -20) -> (90, -30)
  constraint horizontal L32
  constraint vertical L33
  constraint horizontal L34
  constraint vertical L35
extrude "Extrude30" add sketch "Sketch30" along normal blind 100 contours L32 L33 L34 L35
delete_face "DeleteFace1" 1 faces at (-83.3333, 20, 38.3333)
delete_face "DeleteFace2" 1 faces at (-77.0281, -5.2617, 35)
sketch "Sketch31" plane through (0, 0, 5) normal (0, 0, 1) x (-1, 0, 0)
  arc A0 (100, 35) -> (55, 80) centre (55, 35) ccw
  line L0 (55, 80) -> (55, 75)
  line L1 (55, 75) -> (50, 75)
  line L2 (50, 75) -> (50, 80)
  line L3 (50, 80) -> (-90, 80)
  line L4 (-90, 80) -> (-90, 75)
  line L5 (-90, 75) -> (-95, 75)
  line L6 (-95, 75) -> (-95, 80)
  arc A1 (-95, 80) -> (-100, 75) centre (-95, 75) ccw
  line L7 (-100, 75) -> (-100, -75)
  arc A2 (-100, -75) -> (-95, -80) centre (-95, -75) ccw
  line L8 (-95, -80) -> (-95, -75)
  line L9 (-95, -75) -> (-90, -75)
  line L10 (-90, -75) -> (-90, -80)
  line L11 (-90, -80) -> (50, -80)
  line L12 (50, -80) -> (50, -75)
  line L13 (50, -75) -> (55, -75)
  line L14 (55, -75) -> (55, -80)
  arc A3 (55, -80) -> (100, -35) centre (55, -35) ccw
  line L15 (100, -35) -> (100, 35)
  circle A4 centre (-25, 45) radius 2.5
  circle A5 centre (-25, 35) radius 2.5
  circle A6 centre (-25, -35) radius 2.5
  circle A7 centre (-25, -45) radius 2.5
  line L16 (-80, 60) -> (-80, -60)
  line L17 (-80, -60) -> (45, -60)
  line L18 (45, -60) -> (45, -10)
  line L19 (45, -10) -> (50, -10)
  line L20 (50, -10) -> (50, -65)
  line L21 (50, -65) -> (-85, -65)
  line L22 (-85, -65) -> (-85, 65)
  line L23 (-85, 65) -> (50, 65)
  line L24 (50, 65) -> (50, 10)
  line L25 (50, 10) -> (45, 10)
  line L26 (45, 10) -> (45, 60)
  line L27 (45, 60) -> (-80, 60)
  line L28 (90, -5) -> (86, -5)
  line L29 (86, -5) -> (86, 5)
  line L30 (86, 5) -> (90, 5)
  line L31 (90, 5) -> (90, -5)
  dimension "d95" = 4
  constraint horizontal L28
  constraint vertical L29
  constraint horizontal L30
  constraint vertical L31
  measures "d95" distance of L28.start L28.end
extrude "Extrude31" add sketch "Sketch31" along normal blind 65 contours L28 L29 L30 L31
